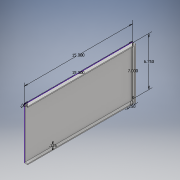
# Autodesk Inventor part: glifPlate
Saved by Autodesk Inventor 2017 (Build 210142000, 142)
## iProperties
Created: 2018-01-06
Part Number: glifPlate
Material: Generic
Document SubType Name: Modeling
Designer: User
Density: 1 g/cm^3
Appearance: Default
Author: User
Autodesk Inventor part; units mm, degrees
ref_plane "YZ Plane" through (0, 0, 0) normal (1, 0, 0) x (0, 1, 0)
ref_plane "XZ Plane" through (0, 0, 0) normal (0, 1, 0) x (-1, 0, 0)
ref_plane "XY Plane" through (0, 0, 0) normal (0, 0, 1) x (1, 0, 0)
sketch "Sketch1" plane through (0, 0, 0) normal (1, 0, 0) x (0, 1, 0)
  line L0 (0, 0) -> (177.8, 0)
  line L1 (177.8, 0) -> (177.8, -381)
  line L2 (177.8, -381) -> (0, -381)
  line L3 (0, -381) -> (0, 0)
  line L4 (3.175, 0) -> (174.625, 0)
  line L5 (174.625, 0) -> (174.625, -381)
  line L6 (174.625, -381) -> (3.175, -381)
  line L7 (3.175, -381) -> (3.175, 0)
  line L8 (177.8, -381) -> (0, -381)
  line L9 (0, -381) -> (0, -374.65)
  line L10 (0, -374.65) -> (177.8, -374.65)
  line L11 (177.8, -374.65) -> (177.8, -381)
  dimension "d0" = 177.8
  dimension "d1" = 381
  dimension "d2" = 171.45
  dimension "d3" = 381
  dimension "d4" = 0
  dimension "d5" = 3.175
  dimension "d10" = 6.35
  constraints: 24 end point, 6 parallel, 3 horizontal, 3 perpendicular, 1 point on line
  measures "d0" distance of L1.end L2.end
  measures "d1" distance of L0.end L1.end
  measures "d2" distance of L5.end L6.end
  measures "d3" distance of L4.end L5.end
  measures "d4" distance between parallel lines of L0 L4
  measures "d5" distance between parallel lines of L3 L7
  measures "d10" distance of L8.end L9.end
extrude "Extrusion1" add sketch "Sketch1" along normal blind 3.175 contours L0 L5 L10 L7 | L10 L5 L2 L7
extrude "Extrusion2" add sketch "Sketch1" along normal blind 12.7 contours L0 L7 L10 L3 | L10 L7 L2 L3 | L0 L1 L10 L5 | L10 L1 L2 L5
extrude "Extrusion3" add sketch "Sketch1" along normal blind 12.7 contours L10 L7 L2 L3 | L10 L5 L2 L7 | L10 L1 L2 L5
body "Solid1"
